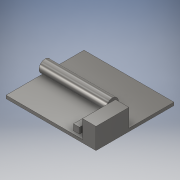
# Autodesk Inventor part: latch
Saved by Autodesk Inventor 2019 (Build 230136000, 136)
## iProperties
Created: 2019-02-16
Part Number: latch
Material: Stainless Steel
Document SubType Name: Modeling
Designer: suchanek
Density: 8 g/cm^3
Appearance: Semi-Polished
Author: suchanek
Autodesk Inventor part; units mm, degrees
ref_plane "YZ Plane" through (0, 0, 0) normal (1, 0, 0) x (0, 1, 0)
ref_plane "XZ Plane" through (0, 0, 0) normal (0, 1, 0) x (-1, 0, 0)
ref_plane "XY Plane" through (0, 0, 0) normal (0, 0, 1) x (1, 0, 0)
sketch "Sketch1" plane through (0, 0, 0) normal (1, 0, 0) x (0, 1, 0)
  line L0 (-0.25, 6.5) -> (0.25, 6.5)
  line L1 (0.25, 6.5) -> (0.25, -6.5)
  line L2 (0.25, -6.5) -> (-0.25, -6.5)
  line L3 (-0.25, -6.5) -> (-0.25, 6.5)
  line L4 (-0.25, 6.5) -> (0.25, -6.5) construction
  line L5 (0.25, 6.5) -> (-0.25, -6.5) construction
  circle A0 centre (1.25, 0) radius 1
  point P0 (0, 0)
  point P1 (0, 0)
  dimension "d0" = 0.5
  dimension "d1" = 13
  dimension "d2" = 2
  constraints: 12 end point, 3 midpoint, 2 parallel, 1 centre point, 1 horizontal, 1 horizontal alignment, 1 perpendicular, 1 tangent
  measures "d0" distance of L1.end L2.end
  measures "d1" distance of L0.end L1.end
  measures "d2" diameter of A0
extrude "Extrusion1" add sketch "Sketch1" along normal blind 15
sketch "Sketch2" plane through (15, 1.25, 0) normal (1, 0, 0) x (0, 0, -1)
  circle A0 centre (0, 0) radius 1
  point P0 (0, -1.25)
  constraints: 1 centre point
extrude "Extrusion2" cut sketch "Sketch2" against normal blind 3.75
sketch "Sketch3" plane through (11.25, 1.25, 0) normal (1, 0, 0) x (0, 0, -1)
  line L0 (0.5, 0.5) -> (-6.5, 0.5)
  line L1 (-6.5, 0.5) -> (-6.5, -0.5)
  line L2 (-6.5, -0.5) -> (0.5, -0.5)
  line L3 (0.5, -0.5) -> (0.5, 0.5)
  line L4 (0.5, 0.5) -> (-6.5, -0.5) construction
  line L5 (-6.5, 0.5) -> (0.5, -0.5) construction
  circle A0 centre (0, 0) radius 1 projected
  line L6 (-6.5, -1) -> (-6.5, -1.5) projected
  point P0 (0, -1.25)
  point P1 (-3, 0)
  point P2 (0, -1)
  point P3 (-3, 0)
  dimension "d11" = 0.5
  dimension "d12" = 1
  dimension "d7" = 0.5
  dimension "d8" = 1
  constraints: 12 end point, 3 midpoint, 2 parallel, 1 coincident, 1 collinear, 1 horizontal, 1 horizontal alignment, 1 perpendicular, 1 vertical alignment
  measures "d7" distance from line of L3 point (0, 0)
  measures "d8" distance of L2.end L0.start
extrude "Extrusion3" add sketch "Sketch3" along normal blind 1 contours L3 L2 A0 L0 | A0 L2 L1 L0 picked at (0.0018, -0.0348)
sketch "Sketch4" plane through (0, 0.25, 6.5) normal (0, 1, 0) x (1, 0, 0)
  line L0 (15, 13) -> (15, 0) projected
  line L1 (15, 0) -> (12.75, 0)
  line L2 (12.75, 0) -> (12.75, 5.5)
  line L3 (12.75, 5.5) -> (15, 5.5)
  line L4 (15, 5.5) -> (15, 0)
  line L5 (12.25, 7) -> (12.25, 0) projected
  line L6 (0, 6.5) -> (11.25, 6.5) projected
  dimension "d11" = 0.5
  dimension "d12" = 1
  constraints: 8 end point, 2 parallel, 1 horizontal, 1 perpendicular
  measures "d11" distance between parallel lines of L5 L2
  measures "d12" distance between parallel lines of L6 L3
extrude "Extrusion4" add sketch "Sketch4" along normal blind 3
body "Solid1"
